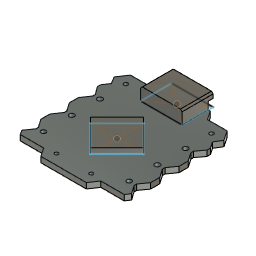
three_knobs_keyboard (Autodesk Fusion 360 archive; units mm, degrees)
design "dfrobot_beetle"
Autodesk Fusion 360 part; units mm, degrees
sketch "Sketch1" plane through (0, 0, 0) normal (0, 0, 1) x (1, 0, 0)
  line L0 (0, 0) -> (120, 0)
  line L1 (120, 0) -> (120, 60)
  line L2 (120, 60) -> (0, 60)
  line L3 (0, 60) -> (0, 0)
  dimension "d1" = 120
  dimension "d2" = 60
  constraint horizontal L0
  constraint vertical L1
  constraint horizontal L2
  constraint vertical L3
  constraint coincident L0.start L3.end
  measures "d1" distance of L0.start L0.end
  measures "d2" distance of L0.start L2.end
extrude "Extrude1" add sketch "Sketch1" along normal blind 10 makes body 1
shell "Shell1" thickness 2 removed faces 1 at (40, 20, 10) on bodies 1
chamfer "Chamfer1" distance 3 angle 45 4 edges at (2, 58, 6) (118, 58, 6) (2, 2, 6) (118, 2, 6) on bodies 1
fillet "Fillet1" radius 3.5 8 edges at (2, 5, 6) (5, 2, 6) (115, 2, 6) (118, 5, 6) (118, 55, 6) (115, 58, 6) (5, 58, 6) (2, 55, 6) on bodies 1
sketch "Sketch1 (2)" plane through (0, 0, 0) normal (0, 0, 1) x (1, 0, 0) in component "beetle_board"
  line L0 (0, 11.4) -> (4.2, 11.4)
  line L1 (4.2, 11.4) -> (5.3, 9.8)
  line L2 (5.3, 9.8) -> (8.9, 9.8)
  line L3 (8.9, 9.8) -> (10.1, 8)
  line L4 (10.1, 8) -> (9.3, 6.7)
  line L5 (9.3, 6.7) -> (10.1, 5.5364)
  line L6 (10.1, 5.5364) -> (10.1, 4.9)
  line L7 (10.1, 4.9) -> (9.035, 3.481)
  line L8 (9.035, 3.481) -> (9.035, 3)
  line L9 (9.035, 3) -> (10.1, 1.4334)
  line L10 (10.1, 1.4334) -> (10.1, -0.2538)
  line L11 (10.1, -0.2538) -> (9.035, -1.7573)
  line L12 (9.035, -1.7573) -> (9.035, -2.25)
  line L13 (9.035, -2.25) -> (10.1, -3.8)
  line L14 (10.1, -3.8) -> (10.1, -5.5)
  line L15 (10.1, -5.5) -> (9.035, -6.9826)
  line L16 (9.035, -6.9826) -> (9.035, -7.4692)
  line L17 (9.035, -7.4692) -> (10.1, -8.9776)
  line L18 (10.1, -8.9776) -> (9.5675, -9.8011)
  line L19 (9.5675, -9.8011) -> (5.25, -9.8011)
  line L20 (5.25, -9.8011) -> (4.1787, -11.3908)
  line L21 (4.1787, -11.3908) -> (0, -11.3908)
  circle A0 centre (7.878, 7.9505) radius 0.3668
  circle A1 centre (7.878, 3.1799) radius 0.4655
  circle A2 centre (7.878, -2.0097) radius 0.4668
  circle A3 centre (7.878, -7.2117) radius 0.4322
  circle A4 centre (3.2, -9.5) radius 0.3291
  line L22 (0, 15) -> (0, -15) construction
  line L23 (-10.1, 1.4334) -> (-10.1, -0.2538)
  line L24 (-10.1, -3.8) -> (-10.1, -5.5)
  line L25 (-10.1, -0.2538) -> (-9.035, -1.7573)
  line L26 (-9.035, -6.9826) -> (-9.035, -7.4692)
  line L27 (-5.3, 9.8) -> (-8.9, 9.8)
  line L28 (-9.035, -1.7573) -> (-9.035, -2.25)
  circle A5 centre (-7.878, -7.2117) radius 0.4322
  line L29 (-9.035, -7.4692) -> (-10.1, -8.9776)
  line L30 (-9.035, -2.25) -> (-10.1, -3.8)
  line L31 (-10.1, -8.9776) -> (-9.5675, -9.8011)
  circle A6 centre (-7.878, 7.9505) radius 0.3668
  line L32 (-10.1, 8) -> (-9.3, 6.7)
  line L33 (0, 11.4) -> (-4.2, 11.4)
  line L34 (-10.1, 5.5364) -> (-10.1, 4.9)
  line L35 (-9.035, 3.481) -> (-9.035, 3)
  line L36 (-4.1787, -11.3908) -> (0, -11.3908)
  line L37 (-9.035, 3) -> (-10.1, 1.4334)
  line L38 (-4.2, 11.4) -> (-5.3, 9.8)
  line L39 (-10.1, 4.9) -> (-9.035, 3.481)
  line L40 (-8.9, 9.8) -> (-10.1, 8)
  line L41 (-9.5675, -9.8011) -> (-5.25, -9.8011)
  line L42 (-10.1, -5.5) -> (-9.035, -6.9826)
  circle A7 centre (-7.878, 3.1799) radius 0.4655
  line L43 (-9.3, 6.7) -> (-10.1, 5.5364)
  line L44 (-5.25, -9.8011) -> (-4.1787, -11.3908)
  circle A8 centre (-3.2, -9.5) radius 0.3291
  circle A9 centre (-7.878, -2.0097) radius 0.4668
  constraint horizontal L0
  constraint parallel L0 L2
  constraint parallel L1 L5
  constraint perpendicular L2 L6
  constraint parallel L6 L8
  constraint parallel L8 L10
  constraint parallel L10 L12
  constraint parallel L12 L14
  constraint parallel L14 L16
  constraint perpendicular L14 L19
  constraint parallel L19 L21
  constraint perpendicular L21 L22
  constraint symmetric L0.start L22 L33.start
  constraint symmetric L0.end L22 L33.end
  constraint symmetric L1.end L22 L27.start
  constraint symmetric L2.end L22 L27.end
  constraint symmetric L3.end L22 L32.start
  constraint symmetric L4.end L22 L32.end
  constraint symmetric L5.end L22 L34.start
  constraint symmetric L6.end L22 L34.end
  constraint symmetric L7.end L22 L35.start
  constraint symmetric L8.end L22 L35.end
  constraint symmetric L9.end L22 L23.start
  constraint symmetric L10.end L22 L23.end
  constraint symmetric L11.end L22 L25.end
  constraint symmetric L12.end L22 L28.end
  constraint symmetric L13.end L22 L24.start
  constraint symmetric L14.end L22 L24.end
  constraint symmetric L15.end L22 L26.start
  constraint symmetric L16.end L22 L26.end
  constraint symmetric L17.end L22 L29.end
  constraint symmetric L18.end L22 L31.end
  constraint symmetric L19.end L22 L41.end
  constraint symmetric L20.end L22 L36.start
  constraint symmetric L21.end L22 L36.end
  constraint symmetric A0 L22 A6
  constraint symmetric A1 L22 A7
  constraint symmetric A2 L22 A9
  constraint symmetric A3 L22 A5
  constraint symmetric A4 L22 A8
extrude "Extrude1'" add sketch "Sketch1 (2)" along normal blind 1.02 separate body makes body 2 in component "beetle_board"
sketch "Sketch2" plane through (0, 0, 1.02) normal (0, 0, 1) x (-1, 0, 0) in component "beetle_board"
  circle A0 centre (-7.878, -7.9505) radius 0.3668
  circle A1 centre (7.878, 2.0097) radius 0.4668
  circle A2 centre (3.2, 9.5) radius 0.3291
  circle A3 centre (7.878, -3.1799) radius 0.4655
  circle A4 centre (7.878, -7.9505) radius 0.3668
  circle A5 centre (7.878, 7.2117) radius 0.4322
  circle A6 centre (-3.2, 9.5) radius 0.3291
  circle A7 centre (-7.878, 7.2117) radius 0.4322
  circle A8 centre (-7.878, 2.0097) radius 0.4668
  circle A9 centre (-7.878, -3.1799) radius 0.4655
  line L0 (-4.2, -11.4) -> (4.2, -11.4)
  line L1 (4.2, -11.4) -> (5.3, -9.8)
  line L2 (5.3, -9.8) -> (8.9, -9.8)
  line L3 (8.9, -9.8) -> (10.1, -8)
  line L4 (10.1, -8) -> (9.3, -6.7)
  line L5 (9.3, -6.7) -> (10.1, -5.5364)
  line L6 (10.1, -5.5364) -> (10.1, -4.9)
  line L7 (10.1, -4.9) -> (9.035, -3.481)
  line L8 (9.035, -3.481) -> (9.035, -3)
  line L9 (9.035, -3) -> (10.1, -1.4334)
  line L10 (10.1, -1.4334) -> (10.1, 0.2538)
  line L11 (10.1, 0.2538) -> (9.035, 1.7573)
  line L12 (9.035, 1.7573) -> (9.035, 2.25)
  line L13 (9.035, 2.25) -> (10.1, 3.8)
  line L14 (10.1, 3.8) -> (10.1, 5.5)
  line L15 (10.1, 5.5) -> (9.035, 6.9826)
  line L16 (9.035, 6.9826) -> (9.035, 7.4692)
  line L17 (9.035, 7.4692) -> (10.1, 8.9776)
  line L18 (10.1, 8.9776) -> (9.5675, 9.8011)
  line L19 (9.5675, 9.8011) -> (5.25, 9.8011)
  line L20 (5.25, 9.8011) -> (4.1787, 11.3908)
  line L21 (4.1787, 11.3908) -> (-4.1787, 11.3908)
  line L22 (-4.1787, 11.3908) -> (-5.25, 9.8011)
  line L23 (-5.25, 9.8011) -> (-9.5675, 9.8011)
  line L24 (-9.5675, 9.8011) -> (-10.1, 8.9776)
  line L25 (-10.1, 8.9776) -> (-9.035, 7.4692)
  line L26 (-9.035, 7.4692) -> (-9.035, 6.9826)
  line L27 (-9.035, 6.9826) -> (-10.1, 5.5)
  line L28 (-10.1, 5.5) -> (-10.1, 3.8)
  line L29 (-10.1, 3.8) -> (-9.035, 2.25)
  line L30 (-9.035, 2.25) -> (-9.035, 1.7573)
  line L31 (-9.035, 1.7573) -> (-10.1, 0.2538)
  line L32 (-10.1, 0.2538) -> (-10.1, -1.4334)
  line L33 (-10.1, -1.4334) -> (-9.035, -3)
  line L34 (-9.035, -3) -> (-9.035, -3.481)
  line L35 (-9.035, -3.481) -> (-10.1, -4.9)
  line L36 (-10.1, -4.9) -> (-10.1, -5.5364)
  line L37 (-10.1, -5.5364) -> (-9.3, -6.7)
  line L38 (-9.3, -6.7) -> (-10.1, -8)
  line L39 (-10.1, -8) -> (-8.9, -9.8)
  line L40 (-8.9, -9.8) -> (-5.3, -9.8)
  line L41 (-5.3, -9.8) -> (-4.2, -11.4)
  line L42 (-3.815, -6.6) -> (3.815, -6.6)
  line L43 (3.815, -6.6) -> (3.815, -12.3)
  line L44 (3.815, -12.3) -> (-3.815, -12.3)
  line L45 (-3.815, -12.3) -> (-3.815, -6.6)
  line L46 (-3.815, -6.6) -> (3.815, -12.3) construction
  line L47 (3.815, -6.6) -> (-3.815, -12.3) construction
  line L48 (-4.879, 1.5692) -> (0, 6.4482)
  line L49 (0, 6.4482) -> (4.879, 1.5692)
  line L50 (4.879, 1.5692) -> (0, -3.3099)
  line L51 (0, -3.3099) -> (-4.879, 1.5692)
  line L52 (-4.879, 1.5692) -> (4.879, 1.5692) construction
  line L53 (0, 6.4482) -> (0, -3.3099) construction
  point P0 (0, -9.45)
  point P1 (0, 1.5692)
  dimension "d80" = 7.63
  dimension "d81" = 5.7
  dimension "d82" = 0.9
  dimension "d85" = 6.9
  dimension "d86" = 6.9
  constraint horizontal L42
  constraint perpendicular L42 L43
  constraint parallel L42 L44
  constraint parallel L43 L45
  constraint coincident L46 P0
  constraint coincident L47 P0
  constraint perpendicular L48 L49
  constraint parallel L48 L50
  constraint parallel L49 L51
  constraint coincident L52 P1
  constraint coincident L53 P1
  measures "d80" distance of L43.end L44.end
  measures "d81" distance of L42.end L43.end
  measures "d82" distance of L0 L44
  measures "d85" distance of L49.end L50.end
  measures "d86" distance of L48.end L49.end
extrude "Extrude2" add sketch "Sketch2" along normal blind 1 contours L48 L49 L50 L51 bodies 2 in component "beetle_board"
extrude "Extrude3" add sketch "Sketch2" along normal blind 2.4 contours L0 L42 L43 L45 | L0 L43 L44 L45 bodies 2 in component "beetle_board"
chamfer "Chamfer1'" distance 1.4 angle 45 2 edges at (3.815, 11.85, 1.02) (-3.815, 11.85, 1.02) on bodies 2 in component "beetle_board"
chamfer "Chamfer2" distance 0.3 angle 45 2 edges at (3.815, 9.45, 3.42) (-3.815, 9.45, 3.42) on bodies 2 in component "beetle_board"
component "beetle_board" placed x (1, 0, 0) y (0, 1, 0) z (0, 0, 1) at (0, 0, 0)
equation "d59 = 2.45 mm * 3"
equation "d66 = ( -2.45 * 3 ) * 1 mm"

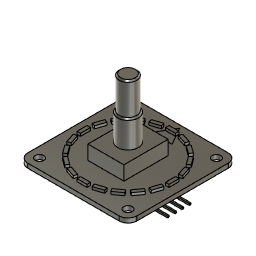
design "dfrobot_knob"
Autodesk Fusion 360 part; units mm, degrees
sketch "Sketch1" plane through (0, 0, 0) normal (0, 0, 1) x (1, 0, 0)
  line L0 (0, 0) -> (120, 0)
  line L1 (120, 0) -> (120, 60)
  line L2 (120, 60) -> (0, 60)
  line L3 (0, 60) -> (0, 0)
  dimension "d1" = 120
  dimension "d2" = 60
  constraint horizontal L0
  constraint vertical L1
  constraint horizontal L2
  constraint vertical L3
  constraint coincident L0.start L3.end
  measures "d1" distance of L0.start L0.end
  measures "d2" distance of L0.start L2.end
extrude "Extrude1" add sketch "Sketch1" along normal blind 10 makes body 1
shell "Shell1" thickness 2 removed faces 1 at (40, 20, 10) on bodies 1
chamfer "Chamfer1" distance 3 angle 45 4 edges at (2, 58, 6) (118, 58, 6) (2, 2, 6) (118, 2, 6) on bodies 1
fillet "Fillet1" radius 3.5 8 edges at (2, 5, 6) (5, 2, 6) (115, 2, 6) (118, 5, 6) (118, 55, 6) (115, 58, 6) (5, 58, 6) (2, 55, 6) on bodies 1
sketch "Sketch1 (2)" plane through (0, 0, 0) normal (0, 0, 1) x (1, 0, 0) in component "rotary_encoder"
  line L0 (18.5, -18.5) -> (-18.5, -18.5)
  line L1 (-18.5, -18.5) -> (-18.5, 18.5)
  line L2 (-18.5, 18.5) -> (18.5, 18.5)
  line L3 (18.5, 18.5) -> (18.5, -18.5)
  line L4 (18.5, -18.5) -> (-18.5, 18.5) construction
  line L5 (-18.5, -18.5) -> (18.5, 18.5) construction
  circle A0 centre (-15, 15) radius 1.45
  circle A1 centre (-15, -15) radius 1.45
  circle A2 centre (15, -15) radius 1.45
  circle A3 centre (15, 15) radius 1.45
  line L6 (6.1, -7.5) -> (-6.1, -7.5)
  line L7 (-6.1, -7.5) -> (-6.1, 7.5)
  line L8 (-6.1, 7.5) -> (6.1, 7.5)
  line L9 (6.1, 7.5) -> (6.1, -7.5)
  line L10 (6.1, -7.5) -> (-6.1, 7.5) construction
  line L11 (-6.1, -7.5) -> (6.1, 7.5) construction
  circle A4 centre (0, 0) radius 3.5
  dimension "d9" = 37
  dimension "d10" = 37
  dimension "d11" = 2.9
  dimension "d12" = 3.5
  dimension "d13" = 3.5
  dimension "d15" = 360
  dimension "d16" = 12.2
  dimension "d17" = 15
  dimension "d18" = 7
  constraint horizontal L0
  constraint perpendicular L0 L1
  constraint parallel L0 L2
  constraint parallel L1 L3
  constraint coincident L4 A4.centre
  constraint coincident L5 A4.centre
  constraint coincident A4.centre origin
  constraint horizontal L6
  constraint perpendicular L6 L7
  constraint parallel L6 L8
  constraint parallel L7 L9
  constraint coincident L10 A4.centre
  constraint coincident L11 A4.centre
  measures "d9" distance of L1.end L2.end
  measures "d10" distance of L0.end L1.end
  measures "d11" diameter of A0
  measures "d12" distance of L1 A0.centre
  measures "d13" distance of L2 A0.centre
  measures "d16" distance of L7.end L8.end
  measures "d17" distance of L6.end L7.end
  measures "d18" diameter of A4
extrude "Extrude1'" add sketch "Sketch1 (2)" along normal blind 1.5 separate body contours L0 L1 L2 L3 makes body 2 in component "rotary_encoder"
extrude "Extrude2" add sketch "Sketch1 (2)" along normal blind 6.3 contours L6 L7 L8 L9 bodies 2 in component "rotary_encoder"
extrude "Extrude3" add sketch "Sketch1 (2)" along normal blind 15.5 contours A4 bodies 2 in component "rotary_encoder"
chamfer "Chamfer1'" distance 0.5 angle 45 1 edges at (-3.2631, -1.2657, 15.5) 1 faces at (0.9018, -0.9121, 15.5) on bodies 2 in component "rotary_encoder"
fillet "Fillet1'" radius 3 4 edges at (18.5, 18.5, 0.75) (18.5, -18.5, 0.75) (-18.5, -18.5, 0.75) (-18.5, 18.5, 0.75) on bodies 2 in component "rotary_encoder"
extrude "Extrude4" add 1 faces at (0.3505, -0.866, 15.5) along direction (0, 0, 1) blind 10.8 on bodies 2 bodies 2 in component "rotary_encoder"
chamfer "Chamfer2" distance 0.5 angle 45 1 edges at (-2.797, -1.0848, 26.3) on bodies 2 in component "rotary_encoder"
sketch "Sketch2" plane through (0, 0, 0) normal (0, 0, 1) x (1, 0, 0) in component "rotary_encoder"
  line L0 (-18.5, -6) -> (-10, -6)
  line L1 (-10, -6) -> (-10, 6)
  line L2 (-10, 6) -> (-18.5, 6)
  line L3 (-18.5, 6) -> (-18.5, -6)
  line L4 (-18.5, -6) -> (-10, 6) construction
  line L5 (-10, -6) -> (-18.5, 6) construction
  line L6 (-18.5, -15.5) -> (-18.5, 15.5)
  line L7 (8.43, -4.9306) -> (10.86, -4.9306)
  line L8 (10.86, -4.9306) -> (10.86, 4.8894)
  line L9 (10.86, 4.8894) -> (8.43, 4.8894)
  line L10 (8.43, 4.8894) -> (8.43, -4.9306)
  line L11 (8.43, -4.9306) -> (10.86, 4.8894) construction
  line L12 (10.86, -4.9306) -> (8.43, 4.8894) construction
  line L13 (18.5, 15.5) -> (18.5, -15.5)
  point P0 (-14.25, 0)
  point P1 (9.645, -0.0206)
  dimension "d31" = 8.5
  dimension "d32" = 12
  dimension "d33" = 8.5
  dimension "d34" = 2.43
  dimension "d35" = 9.82
  dimension "d36" = 10.07
  constraint horizontal L0
  constraint perpendicular L0 L1
  constraint parallel L0 L2
  constraint parallel L1 L3
  constraint coincident L4 P0
  constraint coincident L5 P0
  constraint horizontal L7
  constraint perpendicular L7 L8
  constraint parallel L7 L9
  constraint parallel L8 L10
  constraint coincident L11 P1
  constraint coincident L12 P1
  measures "d31" distance of L1.end L2.end
  measures "d32" distance of L0.end L1.end
  measures "d33" distance of L1 L6
  measures "d34" distance of L8.end L9.end
  measures "d35" distance of L7.end L8.end
  measures "d36" distance of L10 L13
extrude "Extrude5" add sketch "Sketch2" against normal blind 5.68 contours L0 L1 L2 L3 L6 bodies 2 in component "rotary_encoder"
extrude "Extrude6" add sketch "Sketch2" against normal blind 3.16 contours L7 L8 L9 L10 bodies 2 in component "rotary_encoder"
sketch "Sketch3" plane through (0, 0, 1.5) normal (0, 0, 1) x (-1, 0, 0) in component "rotary_encoder"
  circle A0 centre (15, 15) radius 1.45
  circle A1 centre (-15, 15) radius 1.45
  circle A2 centre (-15, -15) radius 1.45
  line L0 (6.1, -7.5) -> (-6.1, -7.5)
  line L1 (-6.1, -7.5) -> (-6.1, 7.5)
  line L2 (-6.1, 7.5) -> (6.1, 7.5)
  line L3 (6.1, 7.5) -> (6.1, -7.5)
  circle A3 centre (15, -15) radius 1.45
  arc A4 (15.5, -18.5) -> (18.5, -15.5) centre (15.5, -15.5) ccw
  line L4 (18.5, -15.5) -> (18.5, 15.5)
  arc A5 (18.5, 15.5) -> (15.5, 18.5) centre (15.5, 15.5) ccw
  line L5 (15.5, 18.5) -> (-15.5, 18.5)
  arc A6 (-15.5, 18.5) -> (-18.5, 15.5) centre (-15.5, 15.5) ccw
  line L6 (-18.5, 15.5) -> (-18.5, -15.5)
  arc A7 (-18.5, -15.5) -> (-15.5, -18.5) centre (-15.5, -15.5) ccw
  line L7 (-15.5, -18.5) -> (15.5, -18.5)
  line L8 (-0.0115, -17.5) -> (3.4698, -11.5099)
  line L9 (3.4698, -11.5099) -> (-3.4584, -11.4901)
  line L10 (-3.4584, -11.4901) -> (-0.0115, -17.5)
  point P0 (0, -13.5)
  dimension "d41" = 2
  measures "d41" distance of P0 L10
extrude "Extrude7" add sketch "Sketch3" along normal blind 0.01 contours L8 L9 L10 bodies 2 in component "rotary_encoder"
sketch "Sketch4" plane through (0, 0, -3.16) normal (0, 0, -1) x (1, 0, 0) in component "rotary_encoder"
  line L0 (8.43, 4.9306) -> (8.43, -4.8894)
  line L1 (8.43, -4.8894) -> (10.86, -4.8894)
  line L2 (10.86, -4.8894) -> (10.86, 4.9306)
  line L3 (10.86, 4.9306) -> (8.43, 4.9306)
  line L4 (10.86, -4.8894) -> (6.1254, -4.8894) construction
  line L5 (10.86, -3.6644) -> (6.1254, -3.6644) construction
  line L6 (10.86, -2.4394) -> (6.1254, -2.4394) construction
  line L7 (10.86, -1.2144) -> (6.1254, -1.2144) construction
  line L8 (10.86, 0.0106) -> (6.1254, 0.0106) construction
  line L9 (10.86, 1.2356) -> (6.1254, 1.2356) construction
  line L10 (10.86, 2.4606) -> (6.1254, 2.4606) construction
  line L11 (10.86, 3.6856) -> (6.1254, 3.6856) construction
  line L12 (10.86, 4.9106) -> (6.1254, 4.9106) construction
  line L13 (9.645, -4.8894) -> (9.645, 4.9306) construction
  line L14 (9.38, -3.3994) -> (9.91, -3.3994)
  line L15 (9.91, -3.3994) -> (9.91, -3.9294)
  line L16 (9.91, -3.9294) -> (9.38, -3.9294)
  line L17 (9.38, -3.9294) -> (9.38, -3.3994)
  line L18 (9.38, -3.3994) -> (9.91, -3.9294) construction
  line L19 (9.91, -3.3994) -> (9.38, -3.9294) construction
  line L20 (9.38, -1.4794) -> (9.38, -0.9494)
  line L21 (9.38, -0.9494) -> (9.91, -0.9494)
  line L22 (9.91, -1.4794) -> (9.38, -1.4794)
  line L23 (9.91, -0.9494) -> (9.91, -1.4794)
  line L24 (9.38, 0.9706) -> (9.38, 1.5006)
  line L25 (9.38, 1.5006) -> (9.91, 1.5006)
  line L26 (9.91, 0.9706) -> (9.38, 0.9706)
  line L27 (9.91, 1.5006) -> (9.91, 0.9706)
  line L28 (9.38, 3.4206) -> (9.38, 3.9506)
  line L29 (9.38, 3.9506) -> (9.91, 3.9506)
  line L30 (9.91, 3.4206) -> (9.38, 3.4206)
  line L31 (9.91, 3.9506) -> (9.91, 3.4206)
  point P0 (9.645, -3.6644)
  point P1 (9.645, -1.2144)
  point P2 (9.645, 1.2356)
  point P3 (9.645, 3.6856)
  dimension "d46" = 0
  dimension "d47" = 9.8
  dimension "d48" = 0.53
  dimension "d49" = 0.53
  dimension "d58" = 0
  dimension "d59" = 7.35
  constraint coincident L1.end L2.start
  constraint perpendicular L0 L4
  constraint midpoint L1 L13.start
  constraint midpoint L3 L13.end
  constraint horizontal L14
  constraint perpendicular L14 L15
  constraint parallel L14 L16
  constraint parallel L15 L17
  constraint coincident L18 P0
  constraint coincident L19 P0
  constraint coincident L13 P0
  constraint coincident L5 P0
  constraint coincident L7 P1
  constraint coincident L13 P1
  constraint coincident L13 P2
  constraint coincident L9 P2
  constraint coincident L11 P3
  constraint coincident L13 P3
  measures "d48" distance of L15.end L16.end
  measures "d49" distance of L14.end L15.end
extrude "Extrude8" add sketch "Sketch4" along normal blind 2.29 contours L14 L15 L16 L17 | L20 L21 L22 L23 | L24 L25 L26 L27 | L28 L29 L30 L31 bodies 2 in component "rotary_encoder"
sketch "Sketch5" plane through (9.91, 0, 0) normal (1, 0, 0) x (0, 1, 0) in component "rotary_encoder"
  line L0 (3.9294, -3.16) -> (3.3994, -3.16)
  line L1 (3.3994, -3.16) -> (3.3994, -5.45)
  line L2 (3.3994, -5.45) -> (3.9294, -5.45)
  line L3 (3.9294, -5.45) -> (3.9294, -3.16)
  line L4 (3.9294, -5.45) -> (3.3994, -5.45)
  line L5 (3.3994, -5.45) -> (3.3994, -4.92)
  line L6 (3.3994, -4.92) -> (3.9294, -4.92)
  line L7 (3.9294, -4.92) -> (3.9294, -5.45)
  line L8 (0.9494, -4.92) -> (1.4794, -4.92)
  line L9 (1.4794, -4.92) -> (1.4794, -5.45)
  line L10 (0.9494, -5.45) -> (0.9494, -4.92)
  line L11 (1.4794, -5.45) -> (0.9494, -5.45)
  line L12 (-1.5006, -4.92) -> (-0.9706, -4.92)
  line L13 (-0.9706, -4.92) -> (-0.9706, -5.45)
  line L14 (-1.5006, -5.45) -> (-1.5006, -4.92)
  line L15 (-0.9706, -5.45) -> (-1.5006, -5.45)
  line L16 (-3.9506, -4.92) -> (-3.4206, -4.92)
  line L17 (-3.4206, -4.92) -> (-3.4206, -5.45)
  line L18 (-3.9506, -5.45) -> (-3.9506, -4.92)
  line L19 (-3.4206, -5.45) -> (-3.9506, -5.45)
  dimension "d62" = 0.53
  dimension "d63" = 0.53
  dimension "d66" = -7.35
  dimension "d67" = 0
  constraint horizontal L4
  constraint vertical L5
  constraint horizontal L6
  constraint vertical L7
  constraint coincident L2.end L3.start
  measures "d62" distance of L2.end L1.end
  measures "d63" distance of L2.end L6.end
extrude "Extrude9" add sketch "Sketch5" along normal blind 7.5 contours L1 L2 L3 L4 L5 L6 L7 | L8 L9 L10 L11 | L12 L13 L14 L15 | L16 L17 L18 L19 bodies 2 in component "rotary_encoder"
sketch "Sketch6" plane through (0, 0, 1.5) normal (0, 0, 1) x (-1, 0, 0) in component "rotary_encoder"
  line L0 (-3.4584, -11.4901) -> (3.4698, -11.5099)
  line L1 (3.4698, -11.5099) -> (-0.0115, -17.5)
  circle A0 centre (15, 15) radius 1.45
  circle A1 centre (-15, 15) radius 1.45
  circle A2 centre (-15, -15) radius 1.45
  line L2 (6.1, -7.5) -> (-6.1, -7.5)
  line L3 (-6.1, -7.5) -> (-6.1, 7.5)
  line L4 (-6.1, 7.5) -> (6.1, 7.5)
  line L5 (6.1, 7.5) -> (6.1, -7.5)
  circle A3 centre (15, -15) radius 1.45
  arc A4 (15.5, -18.5) -> (18.5, -15.5) centre (15.5, -15.5) ccw
  line L6 (18.5, -15.5) -> (18.5, 15.5)
  arc A5 (18.5, 15.5) -> (15.5, 18.5) centre (15.5, 15.5) ccw
  line L7 (15.5, 18.5) -> (-15.5, 18.5)
  arc A6 (-15.5, 18.5) -> (-18.5, 15.5) centre (-15.5, 15.5) ccw
  line L8 (-18.5, 15.5) -> (-18.5, -15.5)
  arc A7 (-18.5, -15.5) -> (-15.5, -18.5) centre (-15.5, -15.5) ccw
  line L9 (-15.5, -18.5) -> (15.5, -18.5)
  line L10 (-1.6943, -14.4) -> (1.7057, -14.4)
  line L11 (1.7057, -14.4) -> (1.7057, -15.6)
  line L12 (1.7057, -15.6) -> (-1.6943, -15.6)
  line L13 (-1.6943, -15.6) -> (-1.6943, -14.4)
  line L14 (-1.6943, -14.4) -> (1.7057, -15.6) construction
  line L15 (1.7057, -14.4) -> (-1.6943, -15.6) construction
  line L16 (6.4429, -14.3094) -> (3.2093, -15.36)
  line L17 (3.2093, -15.36) -> (2.8385, -14.2188)
  line L18 (2.8385, -14.2188) -> (6.0721, -13.1681)
  line L19 (6.0721, -13.1681) -> (6.4429, -14.3094)
  line L20 (10.5494, -11.6181) -> (7.7988, -13.6165)
  line L21 (7.7988, -13.6165) -> (7.0934, -12.6457)
  line L22 (7.0934, -12.6457) -> (9.8441, -10.6472)
  line L23 (9.8441, -10.6472) -> (10.5494, -11.6181)
  line L24 (13.6233, -7.7895) -> (11.6248, -10.5401)
  line L25 (11.6248, -10.5401) -> (10.654, -9.8348)
  line L26 (10.654, -9.8348) -> (12.6524, -7.0841)
  line L27 (12.6524, -7.0841) -> (13.6233, -7.7895)
  line L28 (15.3636, -3.1984) -> (14.3129, -6.432)
  line L29 (14.3129, -6.432) -> (13.1717, -6.0612)
  line L30 (13.1717, -6.0612) -> (14.2223, -2.8276)
  line L31 (14.2223, -2.8276) -> (15.3636, -3.1984)
  line L32 (15.6, 1.7057) -> (15.6, -1.6943)
  line L33 (15.6, -1.6943) -> (14.4, -1.6943)
  line L34 (14.4, -1.6943) -> (14.4, 1.7057)
  line L35 (14.4, 1.7057) -> (15.6, 1.7057)
  line L36 (14.3094, 6.4429) -> (15.36, 3.2093)
  line L37 (15.36, 3.2093) -> (14.2188, 2.8385)
  line L38 (14.2188, 2.8385) -> (13.1681, 6.0721)
  line L39 (13.1681, 6.0721) -> (14.3094, 6.4429)
  line L40 (11.6181, 10.5494) -> (13.6165, 7.7988)
  line L41 (13.6165, 7.7988) -> (12.6457, 7.0934)
  line L42 (12.6457, 7.0934) -> (10.6472, 9.8441)
  line L43 (10.6472, 9.8441) -> (11.6181, 10.5494)
  line L44 (7.7895, 13.6233) -> (10.5401, 11.6248)
  line L45 (10.5401, 11.6248) -> (9.8348, 10.654)
  line L46 (9.8348, 10.654) -> (7.0841, 12.6524)
  line L47 (7.0841, 12.6524) -> (7.7895, 13.6233)
  line L48 (3.1984, 15.3636) -> (6.432, 14.3129)
  line L49 (6.432, 14.3129) -> (6.0612, 13.1717)
  line L50 (6.0612, 13.1717) -> (2.8276, 14.2223)
  line L51 (2.8276, 14.2223) -> (3.1984, 15.3636)
  line L52 (-1.7057, 15.6) -> (1.6943, 15.6)
  line L53 (1.6943, 15.6) -> (1.6943, 14.4)
  line L54 (1.6943, 14.4) -> (-1.7057, 14.4)
  line L55 (-1.7057, 14.4) -> (-1.7057, 15.6)
  line L56 (-6.4429, 14.3094) -> (-3.2093, 15.36)
  line L57 (-3.2093, 15.36) -> (-2.8385, 14.2188)
  line L58 (-2.8385, 14.2188) -> (-6.0721, 13.1681)
  line L59 (-6.0721, 13.1681) -> (-6.4429, 14.3094)
  line L60 (-10.5494, 11.6181) -> (-7.7988, 13.6165)
  line L61 (-7.7988, 13.6165) -> (-7.0934, 12.6457)
  line L62 (-7.0934, 12.6457) -> (-9.8441, 10.6472)
  line L63 (-9.8441, 10.6472) -> (-10.5494, 11.6181)
  line L64 (-13.6233, 7.7895) -> (-11.6248, 10.5401)
  line L65 (-11.6248, 10.5401) -> (-10.654, 9.8348)
  line L66 (-10.654, 9.8348) -> (-12.6524, 7.0841)
  line L67 (-12.6524, 7.0841) -> (-13.6233, 7.7895)
  line L68 (-15.3636, 3.1984) -> (-14.3129, 6.432)
  line L69 (-14.3129, 6.432) -> (-13.1717, 6.0612)
  line L70 (-13.1717, 6.0612) -> (-14.2223, 2.8276)
  line L71 (-14.2223, 2.8276) -> (-15.3636, 3.1984)
  line L72 (-15.6, -1.7057) -> (-15.6, 1.6943)
  line L73 (-15.6, 1.6943) -> (-14.4, 1.6943)
  line L74 (-14.4, 1.6943) -> (-14.4, -1.7057)
  line L75 (-14.4, -1.7057) -> (-15.6, -1.7057)
  line L76 (-14.3094, -6.4429) -> (-15.36, -3.2093)
  line L77 (-15.36, -3.2093) -> (-14.2188, -2.8385)
  line L78 (-14.2188, -2.8385) -> (-13.1681, -6.0721)
  line L79 (-13.1681, -6.0721) -> (-14.3094, -6.4429)
  line L80 (-11.6181, -10.5494) -> (-13.6165, -7.7988)
  line L81 (-13.6165, -7.7988) -> (-12.6457, -7.0934)
  line L82 (-12.6457, -7.0934) -> (-10.6472, -9.8441)
  line L83 (-10.6472, -9.8441) -> (-11.6181, -10.5494)
  line L84 (-7.7895, -13.6233) -> (-10.5401, -11.6248)
  line L85 (-10.5401, -11.6248) -> (-9.8348, -10.654)
  line L86 (-9.8348, -10.654) -> (-7.0841, -12.6524)
  line L87 (-7.0841, -12.6524) -> (-7.7895, -13.6233)
  line L88 (-3.1984, -15.3636) -> (-6.432, -14.3129)
  line L89 (-6.432, -14.3129) -> (-6.0612, -13.1717)
  line L90 (-6.0612, -13.1717) -> (-2.8276, -14.2223)
  line L91 (-2.8276, -14.2223) -> (-3.1984, -15.3636)
  point P0 (0.0057, -15)
  dimension "d70" = 3.4
  dimension "d71" = 1.2
  dimension "d72" = 2.9
  dimension "d74" = 360
  constraint horizontal L10
  constraint perpendicular L10 L11
  constraint parallel L10 L12
  constraint parallel L11 L13
  constraint coincident L14 P0
  constraint coincident L15 P0
  measures "d70" distance of L11.end L12.end
  measures "d71" distance of L10.end L11.end
  measures "d72" distance of L9 L12
extrude "Extrude10" add sketch "Sketch6" along normal blind 0.9 separate body contours L1 L11 L12 | L1 L10 L11 L12 L13 | L16 L17 L18 L19 | L20 L21 L22 L23 | L24 L25 L26 L27 | L28 L29 L30 L31 | L32 L33 L34 L35 | L36 L37 L38 L39 | L40 L41 L42 L43 | L44 L45 L46 L47 | L48 L49 L50 L51 | L52 L53 L54 L55 | L56 L57 L58 L59 | L60 L61 L62 L63 | L64 L65 L66 L67 | L68 L69 L70 L71 | L72 L73 L74 L75 | L76 L77 L78 L79 | L80 L81 L82 L83 | L84 L85 L86 L87 | L88 L89 L90 L91 makes body 3 at (4.1527, 14.6329, 1.5) makes body 4 at (15.2, -0.5609, 1.5) makes body 5 at (4.04, -14.249, 1.5) makes body 6 at (-11.637, -9.1623, 1.5) makes body 7 at (-12.3099, 8.2361, 1.5) makes body 8 at (-14.2827, 5.2305, 1.5) makes body 9 at (-9.153, -11.6437, 1.5) makes body 10 at (9.1623, -11.637, 1.5) makes body 11 at (14.2792, 5.2414, 1.5) makes body 12 at (-5.1178, 13.8988, 1.5) makes body 13 at (9.3881, 11.9673, 1.5) makes body 14 at (14.6329, -4.1527, 1.5) makes body 15 at (0.5724, -15.2, 1.5) makes body 16 at (-14.2792, -5.2414, 1.5) makes body 17 at (-8.4805, 12.6268, 1.5) makes body 18 at (-14.8, -0.5724, 1.5) makes body 19 at (-4.0291, -14.2525, 1.5) makes body 20 at (11.9673, -9.3881, 1.5) makes body 21 at (12.6268, 8.4805, 1.5) makes body 22 at (0.5609, 14.8, 1.5) in component "rotary_encoder"
component "rotary_encoder" placed x (1, 0, 0) y (0, 1, 0) z (0, 0, 1) at (0, 0, 0)
equation "d59 = 2.45 mm * 3"
equation "d66 = ( -2.45 * 3 ) * 1 mm"
